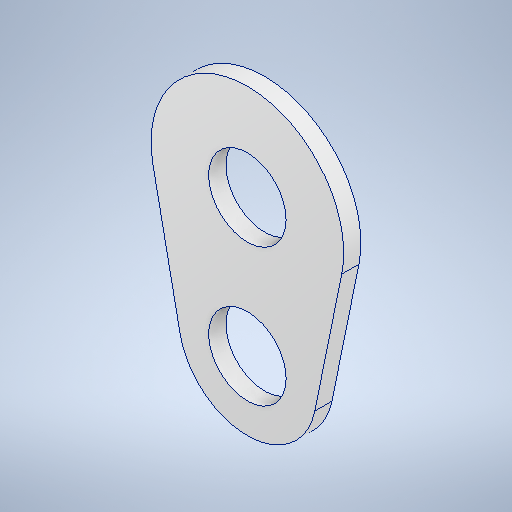
# Autodesk Inventor part: Revised Gearbox Plate #1
Saved by Autodesk Inventor 2025.1 (Build 291241020, 241B)
## iProperties
Created: 2024-09-15
Part Number: Revised Gearbox Plate #1
Material: Aluminum 6061
Document SubType Name: Modeling
Designer: xmand
Density: 2.7 g/cm^3
Appearance: Aluminum - Flat
Author: xmand
Autodesk Inventor part; units mm, degrees
ref_plane "YZ Plane" through (0, 0, 0) normal (1, 0, 0) x (0, 1, 0)
ref_plane "XZ Plane" through (0, 0, 0) normal (0, 1, 0) x (-1, 0, 0)
ref_plane "XY Plane" through (0, 0, 0) normal (0, 0, 1) x (1, 0, 0)
sketch "Sketch1" plane through (0, 0, 0) normal (0, 0, 1) x (1, 0, 0)
  circle A0 centre (0, 0) radius 14.2875
  circle A1 centre (0, 0) radius 20.32 construction
  circle A2 centre (0, 50.8) radius 30.48 construction
  circle A3 centre (0, 50.8) radius 14.2875
  circle A4 centre (0, 50.8) radius 35.56 construction
  circle A5 centre (0, 0) radius 25.4 construction
  line L0 (34.8415, 43.688) -> (24.8868, -5.08)
  line L1 (-34.8415, 43.688) -> (-24.8868, -5.08)
  arc A6 (34.8415, 43.688) -> (-34.8415, 43.688) centre (0, 50.8) ccw
  arc A7 (-24.8868, -5.08) -> (24.8868, -5.08) centre (0, 0) ccw
  dimension "d0" = 28.575
  dimension "d2" = 40.64
  dimension "d6" = 60.96
  dimension "d7" = 28.575
  dimension "d9" = 5.08
  dimension "d10" = 5.08
  constraints: 9 tangent, 8 centre point, 8 point on circle, 5 coincident, 4 end point, 1 vertical alignment
  measures "d0" diameter of A0
  measures "d2" diameter of A1
  measures "d6" diameter of A2
  measures "d7" diameter of A3
  measures "d9" radial gap between concentric circles of A5 A1
  measures "d10" radial gap between concentric circles of A4 A2
extrude "Extrusion1" add sketch "Sketch1" along normal mid plane 6.35
body "Solid1"
